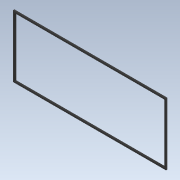
# Autodesk Inventor part: Dichtung_1
Saved by Autodesk Inventor 2020 (Build 240168000, 168)
## iProperties
Created: 2022-02-08
Part Number: Dichtung_1
Material: Gummi
Document SubType Name: Modeling
Designer: Julian Uhl
Density: 0.93 g/cm^3
Appearance: Gummi - Schwarz
Author: Julian Uhl
Autodesk Inventor part; units mm, degrees
ref_plane "YZ Plane" through (0, 0, 0) normal (1, 0, 0) x (0, 1, 0)
ref_plane "XZ Plane" through (0, 0, 0) normal (0, 1, 0) x (-1, 0, 0)
ref_plane "XY Plane" through (0, 0, 0) normal (0, 0, 1) x (1, 0, 0)
sketch "Skizze1" plane through (0, 0, 0) normal (0, 0, 1) x (1, 0, 0)
  line L0 (-55.6, 0) -> (333.6, 0) projected
  line L1 (0, -22.6) -> (0, 135.6) projected
  line L2 (3, 3) -> (275, 3)
  line L3 (275, 3) -> (275, 110)
  line L4 (275, 110) -> (3, 110)
  line L5 (3, 110) -> (3, 3)
  line L6 (0, 0) -> (278, 0)
  line L7 (278, 0) -> (278, 113)
  line L8 (278, 113) -> (0, 113)
  line L9 (0, 113) -> (0, 0)
  point P0 (0, 113)
  point P1 (278, 0)
  dimension "d0" = 272
  dimension "d1" = 107
  dimension "d2" = 3
  dimension "d3" = 3
  dimension "d4" = 3
  dimension "d5" = 3
  constraints: 16 end point, 4 parallel, 2 horizontal, 2 perpendicular
  measures "d0" distance between parallel lines of L3 L5
  measures "d1" distance between parallel lines of L2 L4
  measures "d2" distance between parallel lines of L6 L2
  measures "d3" distance between parallel lines of L9 L5
  measures "d4" distance between parallel lines of L8 L4
  measures "d5" distance between parallel lines of L3 L7
extrude "Extrusion1" add sketch "Skizze1" along normal blind 3
fillet "Rundung1" radius 1 8 edges at (139, 110, 3) (139, 113, 3) (275, 56.5, 3) (278, 56.5, 3) (0, 56.5, 3) (3, 56.5, 3) (139, 3, 3) (139, 0, 3)
